Autodesk Inventor part; units mm, degrees
(part 12 of 12)
  circle A532 centre (-32.385, 14.224) radius 0.2286
  circle A533 centre (-20.32, 18.034) radius 0.2286
  circle A534 centre (-20.32, 18.034) radius 0.2286
  circle A535 centre (-13.111, 7.6) radius 0.2286
  circle A536 centre (-13.111, 7.6) radius 0.2286
  circle A537 centre (-18.7, 37.15) radius 0.2286
  circle A538 centre (-18.7, 37.15) radius 0.2286
  circle A539 centre (-19.676, 22.67) radius 0.2286
  circle A540 centre (-19.676, 22.67) radius 0.2286
  circle A541 centre (-16.3, 38.7) radius 0.2286
  circle A542 centre (-16.3, 38.7) radius 0.2286
  circle A543 centre (-18.149, 21.651) radius 0.2286
  circle A544 centre (-18.149, 21.651) radius 0.2286
  circle A545 centre (-18.7, 38.7) radius 0.2286
  circle A546 centre (-18.7, 38.7) radius 0.2286
  circle A547 centre (-20.322, 20.778) radius 0.2286
  circle A548 centre (-20.322, 20.778) radius 0.2286
  circle A549 centre (-12.78, 35.731) radius 0.2286
  circle A550 centre (-12.78, 35.731) radius 0.2286
  circle A551 centre (-19.5, 37.15) radius 0.2286
  circle A552 centre (-19.5, 37.15) radius 0.2286
  circle A553 centre (-13, 22.3) radius 0.2286
  circle A554 centre (-13, 22.3) radius 0.2286
  circle A555 centre (-13.35, 35) radius 0.2286
  circle A556 centre (-13.35, 35) radius 0.2286
  circle A557 centre (-20.4, 37.15) radius 0.2286
  circle A558 centre (-20.4, 37.15) radius 0.2286
  circle A559 centre (-18.9, 28.573) radius 0.2286
  circle A560 centre (-18.9, 28.573) radius 0.2286
  circle A561 centre (-15.5, 38.7) radius 0.2286
  circle A562 centre (-15.5, 38.7) radius 0.2286
  circle A563 centre (-14.5, 22.3) radius 0.2286
  circle A564 centre (-14.5, 22.3) radius 0.2286
  circle A565 centre (-19.5, 38.7) radius 0.2286
  circle A566 centre (-19.5, 38.7) radius 0.2286
  circle A567 centre (-13.9, 20.7) radius 0.2286
  circle A568 centre (-13.9, 20.7) radius 0.2286
  circle A569 centre (-15.5, 34.925) radius 0.2286
  circle A570 centre (-15.5, 34.925) radius 0.2286
  circle A571 centre (-12.899, 9.58) radius 0.2286
  circle A572 centre (-12.899, 9.58) radius 0.2286
  circle A573 centre (-16.6, 36.65) radius 0.2286
  circle A574 centre (-16.6, 36.65) radius 0.2286
  circle A575 centre (-13.899, 9.58) radius 0.2286
  circle A576 centre (-13.899, 9.58) radius 0.2286
  circle A577 centre (-20.4, 36.4) radius 0.2286
  circle A578 centre (-20.4, 36.4) radius 0.2286
  circle A579 centre (-18.9, 27.273) radius 0.2286
  circle A580 centre (-18.9, 27.273) radius 0.2286
  circle A581 centre (-22.311, 22.097) radius 0.2286
  circle A582 centre (-22.311, 22.097) radius 0.2286
  circle A583 centre (-20.5, 33.1) radius 0.2286
  circle A584 centre (-20.5, 33.1) radius 0.2286
  circle A585 centre (-19.399, 26.384) radius 0.2286
  circle A586 centre (-19.399, 26.384) radius 0.2286
  circle A587 centre (-4.318, 20.701) radius 0.2286
  circle A588 centre (-4.318, 20.701) radius 0.2286
  circle A589 centre (-4.318, 16.764) radius 0.2286
  circle A590 centre (-4.318, 16.764) radius 0.2286
  circle A591 centre (-5.08, 12.827) radius 0.2286
  circle A592 centre (-5.08, 12.827) radius 0.2286
  circle A593 centre (-31.369, 32.512) radius 0.3658
  circle A594 centre (-31.369, 32.512) radius 0.3658
  circle A595 centre (-8.255, 21.717) radius 0.2972
  circle A596 centre (-8.255, 21.717) radius 0.2972
  circle A597 centre (-5.207, 20.701) radius 0.2286
  circle A598 centre (-5.207, 20.701) radius 0.2286
  circle A599 centre (-7.239, 12.827) radius 0.2286
  circle A600 centre (-7.239, 12.827) radius 0.2286
  circle A601 centre (-30.634, 18.515) radius 0.2972
  circle A602 centre (-30.634, 18.515) radius 0.2972
  circle A603 centre (-24.592, 22.079) radius 0.2972
  circle A604 centre (-24.592, 22.079) radius 0.2972
  circle A605 centre (-33.528, 21.717) radius 0.3657
  circle A606 centre (-33.528, 21.717) radius 0.3657
  circle A607 centre (-4.318, 18.161) radius 0.2286
  circle A608 centre (-4.318, 18.161) radius 0.2286
  circle A609 centre (-4.318, 15.113) radius 0.2286
  circle A610 centre (-4.318, 15.113) radius 0.2286
  circle A611 centre (-17.018, 0.635) radius 0.2972
  circle A612 centre (-17.018, 0.635) radius 0.2972
  circle A613 centre (-16.002, 0.635) radius 0.2972
  circle A614 centre (-16.002, 0.635) radius 0.2972
  circle A615 centre (-32.512, 24.638) radius 0.2972
  circle A616 centre (-32.512, 24.638) radius 0.2972
  circle A617 centre (-32.512, 25.4) radius 0.2972
  circle A618 centre (-32.512, 25.4) radius 0.2972
  circle A619 centre (-28.829, 5.461) radius 0.2972
  circle A620 centre (-28.829, 5.461) radius 0.2972
  circle A621 centre (-27.94, 5.461) radius 0.2972
  circle A622 centre (-27.94, 5.461) radius 0.2972
  circle A623 centre (-16.002, 1.397) radius 0.2972
  circle A624 centre (-16.002, 1.397) radius 0.2972
  circle A625 centre (-17.018, 1.397) radius 0.2972
  circle A626 centre (-17.018, 1.397) radius 0.2972
  circle A627 centre (-4.699, 0.635) radius 0.2972
  circle A628 centre (-4.699, 0.635) radius 0.2972
  circle A629 centre (-4.699, 1.524) radius 0.2972
  circle A630 centre (-4.699, 1.524) radius 0.2972
  circle A631 centre (-4.699, 2.413) radius 0.2972
  circle A632 centre (-4.699, 2.413) radius 0.2972
  circle A633 centre (-6.223, 12.827) radius 0.2286
  circle A634 centre (-6.223, 12.827) radius 0.2286
  circle A635 centre (-7.239, 20.701) radius 0.2286
  circle A636 centre (-7.239, 20.701) radius 0.2286
  circle A637 centre (-11.303, 17.653) radius 0.2972
  circle A638 centre (-11.303, 17.653) radius 0.2972
  circle A639 centre (-6.223, 20.701) radius 0.2286
  circle A640 centre (-6.223, 20.701) radius 0.2286
  circle A641 centre (-11.176, 26.289) radius 0.2972
  circle A642 centre (-11.176, 26.289) radius 0.2972
  circle A643 centre (-12.065, 26.289) radius 0.2972
  circle A644 centre (-12.065, 26.289) radius 0.2972
  circle A645 centre (-6.604, 8.509) radius 0.3048
  circle A646 centre (-6.604, 8.509) radius 0.3048
  circle A647 centre (-8.255, 8.509) radius 0.3048
  circle A648 centre (-8.255, 8.509) radius 0.3048
  circle A649 centre (-10.287, 6.477) radius 0.3048
  circle A650 centre (-10.287, 6.477) radius 0.3048
  circle A651 centre (-17.907, 6.477) radius 0.3048
  circle A652 centre (-17.907, 6.477) radius 0.3048
  circle A653 centre (-1.143, 27.051) radius 0.3657
  circle A654 centre (-1.143, 27.051) radius 0.3657
  circle A655 centre (-4.4958, 22.987) radius 0.3657
  circle A656 centre (-4.4958, 22.987) radius 0.3657
  circle A657 centre (-25.527, 26.797) radius 0.3048
  circle A658 centre (-25.527, 26.797) radius 0.3048
  circle A659 centre (-25.527, 5.969) radius 0.3048
  circle A660 centre (-25.527, 5.969) radius 0.3048
  circle A661 centre (-32.512, 26.162) radius 0.2972
  circle A662 centre (-32.512, 26.162) radius 0.2972
  circle A663 centre (-12.192, 4.064) radius 0.2972
  circle A664 centre (-12.192, 4.064) radius 0.2972
  circle A665 centre (-12.192, 1.524) radius 0.2972
  circle A666 centre (-12.192, 1.524) radius 0.2972
  circle A667 centre (-10.414, 1.524) radius 0.2972
  circle A668 centre (-10.414, 1.524) radius 0.2972
  circle A669 centre (-10.414, 4.064) radius 0.2972
  circle A670 centre (-10.414, 4.064) radius 0.2972
  circle A671 centre (-11.303, 4.064) radius 0.2972
  circle A672 centre (-11.303, 4.064) radius 0.2972
  circle A673 centre (-11.303, 1.524) radius 0.2972
  circle A674 centre (-11.303, 1.524) radius 0.2972
  circle A675 centre (-16.873, 41.6) radius 0.2972
  circle A676 centre (-16.873, 41.6) radius 0.2972
  circle A677 centre (-23, 35.1) radius 0.2972
  circle A678 centre (-23, 35.1) radius 0.2972
  circle A679 centre (-22.127, 30.273) radius 0.3657
  circle A680 centre (-22.127, 30.273) radius 0.3657
  circle A681 centre (-18.8, 31.0635) radius 0.2972
  circle A682 centre (-18.8, 31.0635) radius 0.2972
  circle A683 centre (-11.303, 13.208) radius 0.2972
  circle A684 centre (-11.303, 13.208) radius 0.2972
  circle A685 centre (-26.5746, 23.641) radius 0.2286
  circle A686 centre (-26.5746, 23.641) radius 0.2286
  circle A687 centre (-21.209, 30.099) radius 0.2972
  circle A688 centre (-21.209, 30.099) radius 0.2972
  circle A689 centre (-11.176, 25.527) radius 0.2972
  circle A690 centre (-11.176, 25.527) radius 0.2972
  circle A691 centre (-24.638, 40.767) radius 0.3657
  circle A692 centre (-24.638, 40.767) radius 0.3657
  circle A693 centre (-11.811, 35.687) radius 0.3657
  circle A694 centre (-11.811, 35.687) radius 0.3657
  circle A695 centre (-21.59, 9.779) radius 0.2286
  circle A696 centre (-21.59, 9.779) radius 0.2286
  circle A697 centre (-22.479, 9.779) radius 0.2286
  circle A698 centre (-22.479, 9.779) radius 0.2286
  circle A699 centre (-11.303, 14.097) radius 0.2286
  circle A700 centre (-11.303, 14.097) radius 0.2286
  circle A701 centre (-8.071, 29.953) radius 0.2286
  circle A702 centre (-8.071, 29.953) radius 0.2286
  circle A703 centre (-11.303, 14.883) radius 0.2286
  circle A704 centre (-11.303, 14.883) radius 0.2286
  circle A705 centre (-8.071, 30.753) radius 0.2286
  circle A706 centre (-8.071, 30.753) radius 0.2286
  circle A707 centre (-11.303, 15.621) radius 0.2286
  circle A708 centre (-11.303, 15.621) radius 0.2286
  circle A709 centre (-8.071, 31.553) radius 0.2286
  circle A710 centre (-8.071, 31.553) radius 0.2286
  circle A711 centre (-23, 36.7) radius 0.2972
  circle A712 centre (-23, 36.7) radius 0.2972
  circle A713 centre (-3.556, 25.019) radius 0.3657
  circle A714 centre (-3.556, 25.019) radius 0.3657
  circle A715 centre (-2.413, 33.528) radius 0.3657
  circle A716 centre (-2.413, 33.528) radius 0.3657
  circle A717 centre (-20.32, 16.256) radius 0.2286
  circle A718 centre (-20.32, 16.256) radius 0.2286
  circle A719 centre (-29.591, 24.384) radius 0.2286
  circle A720 centre (-29.591, 24.384) radius 0.2286
  circle A721 centre (-19.304, 0.635) radius 0.2972
  circle A722 centre (-19.304, 0.635) radius 0.2972
  circle A723 centre (-19.304, 1.397) radius 0.2972
  circle A724 centre (-19.304, 1.397) radius 0.2972
  circle A725 centre (-18.161, 1.397) radius 0.2972
  circle A726 centre (-18.161, 1.397) radius 0.2972
  circle A727 centre (-18.161, 0.635) radius 0.2972
  circle A728 centre (-18.161, 0.635) radius 0.2972
  circle A729 centre (-30.226, 26.035) radius 0.2286
  circle A730 centre (-30.226, 26.035) radius 0.2286
  circle A731 centre (-21.117, 26.019) radius 0.2286
  circle A732 centre (-21.117, 26.019) radius 0.2286
  circle A733 centre (-29.591, 22.86) radius 0.2286
  circle A734 centre (-29.591, 22.86) radius 0.2286
  circle A735 centre (-26.416, 17.272) radius 0.2286
  circle A736 centre (-26.416, 17.272) radius 0.2286
  circle A737 centre (-29.591, 22.098) radius 0.2286
  circle A738 centre (-29.591, 22.098) radius 0.2286
  circle A739 centre (-26.416, 18.034) radius 0.2286
  circle A740 centre (-26.416, 18.034) radius 0.2286
  circle A741 centre (-22.7838, 26.035) radius 0.2286
  circle A742 centre (-22.7838, 26.035) radius 0.2286
  circle A743 centre (-29.591, 31.115) radius 0.2286
  circle A744 centre (-29.591, 31.115) radius 0.2286
  circle A745 centre (-21.971, 26.035) radius 0.2286
  circle A746 centre (-21.971, 26.035) radius 0.2286
  circle A747 centre (-29.591, 30.353) radius 0.2286
  circle A748 centre (-29.591, 30.353) radius 0.2286
  circle A749 centre (-29.591, 31.9278) radius 0.2286
  circle A750 centre (-29.591, 31.9278) radius 0.2286
  circle A751 centre (-23.622, 26.035) radius 0.2286
  circle A752 centre (-23.622, 26.035) radius 0.2286
  circle A753 centre (-11.303, 11.176) radius 0.2286
  circle A754 centre (-11.303, 11.176) radius 0.2286
  circle A755 centre (-11.303, 12.065) radius 0.2286
  circle A756 centre (-11.303, 12.065) radius 0.2286
  circle A757 centre (-23.78, 22.956) radius 0.2286
  circle A758 centre (-23.78, 22.956) radius 0.2286
  circle A759 centre (-23.876, 13.208) radius 0.2286
  circle A760 centre (-23.876, 13.208) radius 0.2286
  circle A761 centre (-23.876, 13.97) radius 0.2286
  circle A762 centre (-23.876, 13.97) radius 0.2286
  circle A763 centre (-28.956, 10.922) radius 0.2286
  circle A764 centre (-28.956, 10.922) radius 0.2286
  circle A765 centre (-23.876, 14.732) radius 0.2286
  circle A766 centre (-23.876, 14.732) radius 0.2286
  circle A767 centre (-22.098, 5.461) radius 0.2972
  circle A768 centre (-22.098, 5.461) radius 0.2972
  circle A769 centre (-26.797, 8.382) radius 0.2972
  circle A770 centre (-26.797, 8.382) radius 0.2972
  circle A771 centre (-11.303, 19.558) radius 0.2972
  circle A772 centre (-11.303, 19.558) radius 0.2972
  circle A773 centre (-25.527, 23.114) radius 0.2972
  circle A774 centre (-25.527, 23.114) radius 0.2972
  circle A775 centre (-32.512, 27.178) radius 0.2972
  circle A776 centre (-32.512, 27.178) radius 0.2972
  circle A777 centre (-32.512, 28.194) radius 0.2972
  circle A778 centre (-32.512, 28.194) radius 0.2972
  circle A779 centre (-5.715, 6.477) radius 0.2972
  circle A780 centre (-5.715, 6.477) radius 0.2972
  circle A781 centre (-4.699, 6.477) radius 0.2972
  circle A782 centre (-4.699, 6.477) radius 0.2972
  circle A783 centre (-6.731, 6.477) radius 0.2972
  circle A784 centre (-6.731, 6.477) radius 0.2972
  circle A785 centre (-11.176, 24.511) radius 0.2972
  circle A786 centre (-11.176, 24.511) radius 0.2972
  circle A787 centre (-8.255, 17.907) radius 0.2972
  circle A788 centre (-8.255, 17.907) radius 0.2972
  circle A789 centre (-4.318, 32.766) radius 0.2972
  circle A790 centre (-4.318, 32.766) radius 0.2972
  circle A791 centre (-11.176, 23.711) radius 0.2972
  circle A792 centre (-11.176, 23.711) radius 0.2972
  circle A793 centre (-6.731, 5.588) radius 0.2972
  circle A794 centre (-6.731, 5.588) radius 0.2972
  circle A795 centre (-5.715, 5.588) radius 0.2972
  circle A796 centre (-5.715, 5.588) radius 0.2972
  circle A797 centre (-4.953, 8.509) radius 0.3048
  circle A798 centre (-4.953, 8.509) radius 0.3048
  circle A799 centre (-13.843, 6.477) radius 0.3048
  circle A800 centre (-13.843, 6.477) radius 0.3048
  circle A801 centre (-25.527, 9.652) radius 0.3048
  circle A802 centre (-25.527, 9.652) radius 0.3048
  circle A803 centre (-4.699, 3.429) radius 0.2972
  circle A804 centre (-4.699, 3.429) radius 0.2972
  circle A805 centre (-4.699, 4.445) radius 0.2972
  circle A806 centre (-4.699, 4.445) radius 0.2972
  circle A807 centre (-4.699, 5.588) radius 0.2972
  circle A808 centre (-4.699, 5.588) radius 0.2972
  circle A809 centre (-3.302, 32.766) radius 0.2972
  circle A810 centre (-3.302, 32.766) radius 0.2972
  circle A811 centre (-15, 33.1) radius 0.2286
  circle A812 centre (-15, 33.1) radius 0.2286
  circle A813 centre (-26.5746, 22.041) radius 0.2286
  circle A814 centre (-26.5746, 22.041) radius 0.2286
  circle A815 centre (-26.5746, 22.841) radius 0.2286
  circle A816 centre (-26.5746, 22.841) radius 0.2286
  circle A817 centre (-26.5746, 24.441) radius 0.2286
  circle A818 centre (-26.5746, 24.441) radius 0.2286
  circle A819 centre (-26.524, 31.934) radius 0.2286
  circle A820 centre (-26.524, 31.934) radius 0.2286
  circle A821 centre (-26.524, 31.134) radius 0.2286
  circle A822 centre (-26.524, 31.134) radius 0.2286
  circle A823 centre (-26.524, 30.334) radius 0.2286
  circle A824 centre (-26.524, 30.334) radius 0.2286
  circle A825 centre (-26.524, 29.534) radius 0.2286
  circle A826 centre (-26.524, 29.534) radius 0.2286
  circle A827 centre (-33.274, 33.655) radius 0.3657
  circle A828 centre (-33.274, 33.655) radius 0.3657
  circle A829 centre (-23.7, 30.304) radius 0.3657
  circle A830 centre (-23.7, 30.304) radius 0.3657
  circle A831 centre (-21.971, 40.767) radius 0.3657
  circle A832 centre (-21.971, 40.767) radius 0.3657
  circle A833 centre (-8.128, 25.273) radius 0.3657
  circle A834 centre (-8.128, 25.273) radius 0.3657
  circle A835 centre (-12.065, 39.497) radius 0.3657
  circle A836 centre (-12.065, 39.497) radius 0.3657
  constraints: 19822 end point, 10333 symmetric about line, 836 centre point, 12 point on circle, 1 vertical, 418 other
ref_plane "作業平面2" through (-4.4936, -5, 0) normal (0, 0.8660254, 0.5) x (-1, 0, 0)
sketch "スケッチ4" plane through (-4.4936, -5, 0) normal (0, 0.8660254, 0.5) x (-1, 0, 0)
  line L0 (-22.977, 0.2256) -> (0, 0.2256)
  line L1 (-22.977, 0.2256) -> (-22.977, 4.924)
  line L2 (0, 4.924) -> (-22.977, 4.924)
  line L3 (0, 0.2256) -> (0, 4.924)
  line L4 (-45.56, 0.2256) -> (-40.56, 0.2256)
  line L5 (-45.56, 0.2256) -> (-45.56, 4.924)
  line L6 (-40.56, 4.924) -> (-45.56, 4.924)
  line L7 (-40.56, 0.2256) -> (-40.56, 4.924)
  line L8 (-45.56, 4.924) -> (-45.56, -20.076)
  line L9 (-45.56, -20.076) -> (0, -20.076)
  line L10 (0, -20.076) -> (0, 4.924)
  line L11 (-22.977, 0.2256) -> (-22.977, 4.924)
  line L12 (-40.56, 4.924) -> (-40.56, -7.076)
  line L13 (-40.56, -7.076) -> (-22.977, -7.076)
  line L14 (-22.977, -7.076) -> (-22.977, 4.924)
  line L15 (0, 0) -> (22.78, 0) projected
  line L16 (0, 0) -> (0, 4.924) projected
  line L17 (22.78, 4.924) -> (0, 4.924) projected
  line L18 (22.78, 0) -> (22.78, 4.924) projected
  line L19 (0, 4.924) -> (-22.977, 4.924)
  line L20 (-40.56, 4.924) -> (-45.56, 4.924)
  point P0 (-5, -5.5888)
  point P1 (-45.5531, 4.3591)
  constraints: 34 end point, 4 parallel, 2 perpendicular
extrude "押し出し4" add sketch "スケッチ4" along normal blind 3.5 contours L1 L2 L3 L0 | L0 L10 L9 L8 L4 L12 L13 L14 | L4 L5 L6 L7
sketch "スケッチ5" plane through (-4.4936, -5, 0) normal (0, -0.8660254, -0.5) x (1, 0, 0)
  circle A0 centre (4.434, -10.076) radius 1.75
  circle A1 centre (41.06, -16.076) radius 1.75
  circle A2 centre (4.434, -16.076) radius 1.75
  circle A3 centre (41.06, -10.076) radius 1.75
  line L0 (40.5829, -7.076) -> (40.5829, 4.924)
  line L1 (40.5829, -7.076) -> (26.1338, -7.076)
  line L2 (26.1338, -7.076) -> (26.1338, 4.924)
  line L3 (-0.066, 4.924) -> (26.1338, 4.924)
  line L4 (-0.066, -20.076) -> (-0.066, 4.924)
  line L5 (45.56, -20.076) -> (-0.066, -20.076)
  line L6 (45.56, -20.076) -> (45.56, 4.924)
  line L7 (40.5829, 4.924) -> (45.56, 4.924)
  point P0 (-17.78, -1.7365)
  point P1 (21.3541, -0.076)
  point P2 (22.78, -20.3015)
  point P3 (-45.56, 0)
  constraints: 16 end point, 4 centre point
extrude "押し出し5" cut sketch "スケッチ5" against normal blind 5 contours A0 | A1 | A2 | A3
chamfer "面取り2" distance 2 angle 45 2 edges at (38.5629, -0.9585, 0) (6.8964, -0.9585, 0)
sketch "スケッチ7" plane through (0, 0, 5) normal (0, 0, 1) x (1, 0, 0)
  line L0 (-34.4571, 14.3951) -> (74.8417, 14.3951)
  line L1 (74.8417, 14.3951) -> (74.8417, -29.1159)
  line L2 (74.8417, -29.1159) -> (-34.4571, -29.1159)
  line L3 (-34.4571, -29.1159) -> (-34.4571, 14.3951)
  point P0 (0, 0)
  constraints: 8 end point, 2 parallel, 1 horizontal, 1 perpendicular
extrude "押し出し6" cut sketch "スケッチ7" along normal blind 5
chamfer "面取り5" distance 3 angle 45 2 edges at (-4.4936, 47.068, 2.5) (41.0595, 47.01, 2.5)
sketch "スケッチ9" plane through (0, 0, 0) normal (0, 0, -1) x (-1, 0, 0)
  line L0 (-0.94, 31.399) -> (-0.94, 28.799) projected
  line L1 (-1.34, 31.099) -> (-2.34, 31.099) projected
  line L2 (-3.74, 29.099) -> (-2.74, 29.099) projected
  line L3 (-2.34, 31.099) -> (-2.74, 29.099)
  circle A0 centre (-2.54, 30.099) radius 2.5
  point P0 (0, 0)
  dimension "d62" = 5
  constraints: 2 end point, 1 centre point, 1 midpoint
  measures "d62" diameter of A0
extrude "押し出し7" cut sketch "スケッチ9" against normal blind 10
sketch "スケッチ10" plane through (18.2864, -3.8453, 5) normal (1, 0, 0) x (0, 0, -1)
  line L0 (6.6603, 3.8453) -> (0, 0) projected
  line L1 (6.6603, 3.8453) -> (0, 3.8453) projected
  line L2 (0, 0) -> (0, 3.8453) projected
  point P0 (5, 3.8453)
extrude "押し出し8" cut sketch "スケッチ10" against normal blind 18.286
